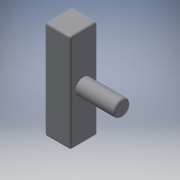
# Autodesk Inventor part: BackWheelMount
Saved by Autodesk Inventor 2018 (Build 220112000, 112)
## iProperties
Created: 2017-11-24
Part Number: BackWheelMount
Material: Generic
Document SubType Name: Modeling
Designer: reide
Density: 1 g/cm^3
Appearance: Default
Author: reide
Autodesk Inventor part; units mm, degrees
ref_plane "YZ Plane" through (0, 0, 0) normal (1, 0, 0) x (0, 1, 0)
ref_plane "XZ Plane" through (0, 0, 0) normal (0, 1, 0) x (-1, 0, 0)
ref_plane "XY Plane" through (0, 0, 0) normal (0, 0, 1) x (1, 0, 0)
sketch "Sketch1" plane through (0, 0, 0) normal (0, 0, 1) x (1, 0, 0)
  line L0 (100.4457, -5.6676) -> (100.4457, -66.5884) projected
  line L1 (75.0457, -66.5884) -> (75.0457, -5.6676) projected
  line L2 (75.0457, -5.6676) -> (55.9957, -5.6676)
  line L3 (55.9957, -5.6676) -> (55.9957, -66.5884)
  line L4 (55.9957, -66.5884) -> (75.0457, -66.5884)
  line L5 (75.0457, -66.5884) -> (75.0457, -5.6676)
  line L6 (75.0457, -5.6676) -> (62.3457, -5.6676)
  line L7 (62.3457, -5.6676) -> (62.3457, -66.5884)
  line L8 (62.3457, -66.5884) -> (75.0457, -66.5884)
  line L9 (75.0457, -66.5884) -> (75.0457, -5.6676)
  line L10 (55.9957, -5.6676) -> (59.1707, -5.6676)
  line L11 (59.1707, -5.6676) -> (59.1707, -66.5884)
  line L12 (59.1707, -5.6676) -> (59.1707, -12.0176)
  circle A0 centre (59.1707, -12.0176) radius 1.5
  line L13 (59.1707, -66.5884) -> (59.1707, -60.2384)
  circle A1 centre (59.1707, -60.2384) radius 1.5
  line L14 (59.1707, -12.0176) -> (59.1707, -36.1222)
  circle A2 centre (59.1707, -36.1222) radius 1.5
  point P0 (0, 0)
  dimension "d0" = 19.05
  dimension "d1" = 12.7
  dimension "d2" = 3.175
  dimension "d3" = 6.35
  dimension "d4" = 3
  dimension "d5" = 6.35
  dimension "d6" = 3
  dimension "d7" = 24.1046
  dimension "d8" = 3
  constraints: 26 end point, 6 point on line, 4 parallel, 3 centre point, 3 coincident, 3 perpendicular, 2 horizontal
  measures "d0" distance of L3.end L4.end
  measures "d1" distance of L8.end L7.end
  measures "d2" distance of L2.end L10.end
  measures "d3" distance of L10.end L12.end
  measures "d4" diameter of A0
  measures "d5" distance of L11.end L13.end
  measures "d6" diameter of A1
  measures "d7" distance of L14.start L14.end
  measures "d8" diameter of A2
extrude "Extrusion1" add sketch "Sketch1" along normal blind 12.7
sketch "Sketch2" plane through (75.0457, -66.5884, 0) normal (1, 0, 0) x (0, 0, -1)
  line L0 (0, 60.9208) -> (0, 0) projected
  line L1 (0, 0) -> (0, 30.4546)
  line L2 (0, 30.4546) -> (-6.35, 30.4546)
  circle A0 centre (-6.35, 30.4546) radius 3.95
  point P0 (0, 66.5884)
  dimension "d11" = 30.4546
  dimension "d12" = 6.35
  dimension "d13" = 7.9
  constraints: 4 end point, 1 centre point, 1 coincident, 1 perpendicular, 1 point on line
  measures "d11" distance of L0.end L1.end
  measures "d12" distance of L1.end L2.end
  measures "d13" diameter of A0
extrude "Extrusion2" add sketch "Sketch2" along normal blind 19.05
sketch "Sketch3" plane through (0, 0, 12.7) normal (0, 0, 1) x (1, 0, 0)
  line L0 (75.0457, -5.6676) -> (55.9957, -5.6676)
  line L1 (55.9957, -5.6676) -> (55.9957, -66.5884)
  line L2 (55.9957, -66.5884) -> (75.0457, -66.5884)
  line L3 (75.0457, -5.6676) -> (62.3457, -5.6676)
  line L4 (62.3457, -5.6676) -> (62.3457, -66.5884)
  line L5 (62.3457, -66.5884) -> (75.0457, -66.5884)
  line L6 (55.9957, -5.6676) -> (59.1707, -5.6676)
  line L7 (59.1707, -5.6676) -> (59.1707, -66.5884)
  line L8 (59.1707, -5.6676) -> (59.1707, -12.0176)
  circle A0 centre (59.1707, -12.0176) radius 1.5
  line L9 (59.1707, -66.5884) -> (59.1707, -60.2384)
  circle A1 centre (59.1707, -60.2384) radius 1.5
  line L10 (59.1707, -12.0176) -> (59.1707, -36.1222)
  circle A2 centre (59.1707, -36.1222) radius 1.5
  line L11 (55.9957, -5.6676) -> (62.3457, -5.6676)
  line L12 (62.3457, -5.6676) -> (62.3457, -66.5884)
  line L13 (62.3457, -66.5884) -> (55.9957, -66.5884)
  line L14 (55.9957, -66.5884) -> (55.9957, -5.6676)
  line L15 (75.0457, -66.5884) -> (75.0457, -5.6676) projected
  line L16 (62.3457, -5.6676) -> (75.0457, -5.6676)
  line L17 (75.0457, -5.6676) -> (75.0457, -12.0176)
  line L18 (75.0457, -12.0176) -> (62.3457, -12.0176)
  line L19 (62.3457, -12.0176) -> (62.3457, -5.6676)
  line L20 (62.3457, -66.5884) -> (75.0457, -66.5884)
  line L21 (75.0457, -66.5884) -> (75.0457, -60.2384)
  line L22 (75.0457, -60.2384) -> (62.3457, -60.2384)
  line L23 (62.3457, -60.2384) -> (62.3457, -66.5884)
  point P0 (0, 0)
  dimension "d16" = 19.05
  dimension "d17" = 12.7
  dimension "d18" = 3.175
  dimension "d19" = 6.35
  dimension "d20" = 3
  dimension "d21" = 6.35
  dimension "d22" = 3
  dimension "d23" = 24.1046
  dimension "d24" = 3
  dimension "d27" = 60.9208
  dimension "d28" = 6.35
  dimension "d29" = 6.35
  constraints: 46 end point, 8 parallel, 8 point on line, 6 perpendicular, 5 horizontal, 3 centre point, 3 coincident
  measures "d16" distance of L1.end L2.end
  measures "d17" distance of L5.end L4.end
  measures "d18" distance of L1.start L7.start
  measures "d19" distance of L7.start L8.end
  measures "d20" diameter of A0
  measures "d21" distance of L7.end L9.end
  measures "d22" diameter of A1
  measures "d23" distance of L10.start L10.end
  measures "d24" diameter of A2
  measures "d27" distance of L2.end L0.start
  measures "d28" distance between parallel lines of L18 L3
  measures "d29" distance between parallel lines of L2 L22
extrude "Extrusion3" cut sketch "Sketch3" against normal blind 2540 contours L15 L18 L4 L0 | L4 L2 L7 A1 A2 A0 L0 | L7 A0 A2 A1 L2 L1 L0 | L15 L2 L4 L22 | A0 L7 | L7 A0 | A2 L7 | L7 A2 | A1 L7 | L7 A1
fillet "Fillet1" radius 1 8 edges at (62.3457, -36.128, 12.7) (75.0457, -36.128, 12.7) (68.6957, -60.2384, 12.7) (68.6957, -12.0176, 12.7) (62.3457, -12.0176, 6.35) (62.3457, -60.2384, 6.35) (75.0457, -60.2384, 6.35) (75.0457, -12.0176, 6.35)
fillet "Fillet2" radius 1 1 edges at (94.0957, -36.1338, 10.3)
fillet "Fillet3" [suppressed]
sketch "Sketch5" plane through (0, 0, 0) normal (0, 0, -1) x (-1, 0, 0)
  line L0 (-63.3457, -12.0176) -> (-74.0457, -12.0176) projected
  line L1 (-74.0457, -12.0176) -> (-72.0457, -12.0176)
  line L2 (-72.0457, -12.0176) -> (-72.0457, -15.0176)
  circle A0 centre (-72.0457, -15.0176) radius 1.25
  line L3 (-68.6957, -12.0176) -> (-68.6957, -9.3578)
  line L4 (-62.3457, -59.2384) -> (-62.3457, -13.0176) projected
  line L5 (-62.3457, -36.128) -> (-58.1504, -36.128)
  line L6 (-74.0457, -12.0176) -> (-63.3457, -12.0176)
  line L7 (-63.3457, -12.0176) -> (-65.3457, -12.0176)
  line L8 (-65.3457, -12.0176) -> (-65.3457, -15.0176)
  circle A1 centre (-65.3457, -15.0176) radius 1.25
  line L9 (-72.0457, -60.2384) -> (-72.0457, -57.2384)
  circle A2 centre (-72.0457, -57.2384) radius 1.25
  line L10 (-65.3457, -60.2384) -> (-65.3457, -57.2384)
  circle A3 centre (-65.3457, -57.2384) radius 1.25
  point P0 (0, 0)
  dimension "d48" = 2
  dimension "d49" = 3
  dimension "d50" = 2.5
  constraints: 18 end point, 11 symmetric about line, 4 centre point, 4 coincident, 2 midpoint, 2 point on line, 1 horizontal, 1 perpendicular, 1 vertical, 3 other
  measures "d48" distance of L0.end L1.end
  measures "d49" distance of L1.end L2.end
  measures "d50" diameter of A0
extrude "Extrusion5" cut sketch "Sketch5" against normal blind 9
body "Solid1"
